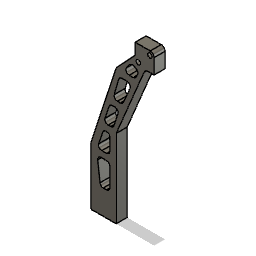
arma_1_(version_minecraft)_v3 (Autodesk Fusion 360 design; units mm, degrees)
Autodesk Fusion 360 part; units mm, degrees
sketch "Boceto1" plane through (0, 0, 0) normal (0, 0, 1) x (1, 0, 0)
sketch "Boceto2" plane through (0, 0, 0) normal (0, 0, 1) x (1, 0, 0)
  line L0 (0, 0) -> (0, 77.2995)
  line L1 (0, 77.2995) -> (40, 200)
  line L2 (40, 200) -> (77.2455, 240)
  line L3 (77.2455, 240) -> (94.1667, 240)
  line L4 (94.1667, 240) -> (40, 110)
  line L5 (40, 110) -> (40, 0)
  line L6 (40, 0) -> (0, 0)
  line L7 (73, 230) -> (85, 230)
  line L8 (85, 230) -> (70, 200)
  line L9 (70, 200) -> (50, 200)
  line L10 (50, 200) -> (73, 230)
  line L11 (45, 190) -> (65, 190)
  line L12 (65, 190) -> (50, 155)
  line L13 (50, 155) -> (35, 155)
  line L14 (35, 155) -> (45, 190)
  line L15 (30, 145) -> (45, 145)
  line L16 (45, 145) -> (35, 115)
  line L17 (35, 115) -> (20, 115)
  line L18 (20, 115) -> (30, 145)
  line L19 (20, 105) -> (30, 105)
  line L20 (30, 105) -> (30, 75)
  line L21 (30, 75) -> (10, 75)
  line L22 (10, 75) -> (20, 105)
  line L23 (10, 65) -> (30, 65)
  line L24 (30, 65) -> (30, 25)
  line L25 (30, 25) -> (15, 25)
  line L26 (15, 25) -> (10, 65)
  constraint coincident L0.start L6.end
  constraint vertical L0
  constraint perpendicular L0 L3
  constraint vertical L5
  constraint perpendicular L0 L6
  constraint horizontal L7
  constraint parallel L7 L9
  constraint horizontal L11
  constraint parallel L11 L13
  constraint horizontal L15
  constraint parallel L15 L17
  constraint parallel L16 L18
  constraint horizontal L19
  constraint perpendicular L19 L20
  constraint perpendicular L20 L21
  constraint horizontal L23
  constraint perpendicular L23 L24
  constraint perpendicular L24 L25
extrude "Extruir1" add sketch "Boceto2" along normal blind 10 makes body 1
cylinder "CilindroPrimitivo1" add diameter 47.743 height 10 placed x (1, 0, 0) y (0, 1, 0) z (0, 0, 1) at (20, 10, 10) separate body makes body 2
copy_body "CopiarPegarCuerpos1" bodies 2 makes body 3
move_body "Desplazar1" bodies 3 to x (1, 0, 0) y (0, 1, 0) z (0, 0, 1) at (0, 0, -20)
hole "Agujero1" at (20.2379, 10.8287, -10) direction (0, 0, 1) diameter 20 depth 20 tip angle 118 bodies 1 2 3
hole "Agujero2" at (20, 10, 20) direction (0, 0, -1) diameter 20 depth 20 tip angle 118 bodies 1 2 3
sketch "Boceto4" plane through (0, 0, 0) normal (0, 0, 1) x (1, 0, 0)
sketch "Boceto5" plane through (0, 0, 10) normal (0, 0, 1) x (1, 0, 0)
  arc A0 (10.5162, 13.1713) -> (20, 0) centre (20, 10) ccw
  arc A1 (29.7218, 7.6575) -> (10.5162, 13.1713) centre (20.2379, 10.8287) ccw
  arc A2 (20, 0) -> (29.7218, 7.6575) centre (20, 10) ccw
  line L0 (20, 0) -> (40, 0)
  line L1 (40, 0) -> (40, 110)
  line L2 (40, 110) -> (94.1667, 240)
  line L3 (94.1667, 240) -> (77.2455, 240)
  line L4 (77.2455, 240) -> (40, 200)
  line L5 (40, 200) -> (0, 77.2995)
  line L6 (0, 77.2995) -> (0, 0)
  line L7 (0, 0) -> (20, 0)
  line L8 (70, 200) -> (50, 200)
  line L9 (50, 200) -> (73, 230)
  line L10 (73, 230) -> (85, 230)
  line L11 (85, 230) -> (70, 200)
  line L12 (50, 155) -> (35, 155)
  line L13 (35, 155) -> (45, 190)
  line L14 (45, 190) -> (65, 190)
  line L15 (65, 190) -> (50, 155)
  line L16 (35, 115) -> (20, 115)
  line L17 (20, 115) -> (30, 145)
  line L18 (30, 145) -> (45, 145)
  line L19 (45, 145) -> (35, 115)
  line L20 (30, 75) -> (10, 75)
  line L21 (10, 75) -> (20, 105)
  line L22 (20, 105) -> (30, 105)
  line L23 (30, 105) -> (30, 75)
  line L24 (30, 25) -> (15, 25)
  line L25 (15, 25) -> (10, 65)
  line L26 (10, 65) -> (30, 65)
  line L27 (30, 65) -> (30, 25)
  line L28 (50, 340) -> (50, 330)
  line L29 (50, 330) -> (60, 330)
  line L30 (60, 330) -> (60, 320)
  line L31 (60, 320) -> (100, 320)
  line L32 (100, 320) -> (100, 310)
  line L33 (100, 310) -> (110, 310)
  line L34 (110, 310) -> (110, 300)
  line L35 (110, 300) -> (120, 300)
  line L36 (120, 300) -> (120, 260)
  line L37 (120, 260) -> (130, 260)
  line L38 (130, 260) -> (130, 250)
  line L39 (130, 250) -> (140, 250)
  line L40 (140, 250) -> (140, 260)
  line L41 (140, 260) -> (150, 260)
  line L42 (150, 260) -> (150, 310)
  line L43 (150, 310) -> (140, 310)
  line L44 (140, 310) -> (140, 340)
  line L45 (140, 340) -> (110, 340)
  line L46 (110, 340) -> (110, 350)
  line L47 (110, 350) -> (60, 350)
  line L48 (60, 350) -> (60, 340)
  line L49 (60, 340) -> (50, 340)
  constraint vertical L28
  constraint perpendicular L28 L29
  constraint perpendicular L29 L30
  constraint perpendicular L30 L31
  constraint perpendicular L29 L32
  constraint perpendicular L32 L33
  constraint perpendicular L33 L34
  constraint perpendicular L34 L35
  constraint perpendicular L35 L36
  constraint perpendicular L36 L37
  constraint perpendicular L37 L38
  constraint perpendicular L38 L39
  constraint perpendicular L39 L40
  constraint perpendicular L40 L41
  constraint perpendicular L41 L42
  constraint perpendicular L42 L43
  constraint perpendicular L43 L44
  constraint perpendicular L44 L45
  constraint perpendicular L43 L46
  constraint perpendicular L46 L47
  constraint perpendicular L47 L48
  constraint perpendicular L28 L49
extrude "Extruir2" add sketch "Boceto5" along normal blind 10 separate body contours L28 L29 L30 L31 L32 L33 L34 L35 L36 L37 L38 L39 L40 L41 L42 L43 L44 L45 L46 L47 L48 L49 makes body 4
move_body "Desplazar2" bodies 4 to x (1, 0, 0) y (0, 1, 0) z (0, 0, 1) at (-20.4494, -47.9195, 22.1569)
move_body "Desplazar3" bodies 4 to x (1, 0, 0) y (0, 1, 0) z (0, 0, 1) at (4.6161, -12.0805, -32.1569)
move_body "Desplazar4" bodies 4 to x (1, 0, 0) y (0, 1, 0) z (0, 0, 1) at (0, -10, 0)
box "CajaPrimitiva1" add length 30 width 30 height 10 placed x (0, -1, 0) y (-1, 0, 0) z (0, 0, -1) at (100, 250, 0) separate body makes body 5
box "CajaPrimitiva2" cut length 30 width 30 height 10 placed x (0, -1, 0) y (1, 0, 0) z (0, 0, 1) at (70, 250, 0) bodies 1 4
move_body "Desplazar6" bodies 5 to x (1, 0, 0) y (0, 1, 0) z (0, 0, 1) at (0, 0, 10)
delete_body "QuitarCuerpo1" bodies 2
delete_body "QuitarCuerpo2" bodies 3
scale "Escala1" factor 0.9 about (40, 110, 0) bodies 4 5 1
scale "Escala2" factor 0.8 about (40, 110, 0) bodies 5 4 1
scale "Scale3" factor 0.8 about (40, 110, 0) bodies 5 4 1
copy_body "CopyPasteBodies3" bodies 1 5 4 makes body 6 makes body 7 makes body 8
sketch "Sketch8" plane through (0, 0, 5.76) normal (0, 0, 1) x (1, 0, 0)
  line L0 (42.4, 190.64) -> (74.56, 190.64)
  line L1 (74.56, 190.64) -> (74.56, 179.12)
  line L2 (74.56, 179.12) -> (76.96, 179.12)
  line L3 (76.96, 179.12) -> (76.96, 156.08)
  line L4 (76.96, 156.08) -> (82.72, 156.08)
  line L5 (82.72, 156.08) -> (82.72, 150.32)
  line L6 (82.72, 150.32) -> (88.48, 150.32)
  line L7 (88.48, 150.32) -> (88.48, 156.08)
  line L8 (88.48, 156.08) -> (94.24, 156.08)
  line L9 (94.24, 156.08) -> (94.24, 184.88)
  line L10 (94.24, 184.88) -> (88.48, 184.88)
  line L11 (88.48, 184.88) -> (88.48, 202.16)
  line L12 (88.48, 202.16) -> (71.2, 202.16)
  line L13 (71.2, 202.16) -> (71.2, 207.92)
  line L14 (71.2, 207.92) -> (42.4, 207.92)
  line L15 (42.4, 207.92) -> (42.4, 202.16)
  line L16 (42.4, 202.16) -> (36.64, 202.16)
  line L17 (36.64, 202.16) -> (36.64, 196.4)
  line L18 (36.64, 196.4) -> (42.4, 196.4)
  line L19 (42.4, 196.4) -> (42.4, 190.64)
  line L20 (57.28, 173.36) -> (74.56, 173.36)
  line L21 (74.56, 173.36) -> (74.56, 190.64)
  line L22 (74.56, 190.64) -> (57.28, 190.64)
  line L23 (57.28, 190.64) -> (57.28, 173.36)
  circle A0 centre (62.9785, 200.1725) radius 2
  line L24 (62.9785, 200.1725) -> (84.1917, 178.9593)
  circle A1 centre (84.1917, 178.9593) radius 2
  circle A2 centre (60.1084, 176.1884) radius 2
  line L25 (60.1084, 176.1884) -> (70.715, 186.795)
  circle A3 centre (70.715, 186.795) radius 2
  line L26 (57.28, 173.36) -> (74.56, 190.64) construction
  dimension "d32" = 4
  dimension "d33" = 30
  dimension "d34" = 4
  dimension "d35" = 4
  dimension "d36" = 15
  dimension "d37" = 4
  dimension "d38" = 5
  dimension "d39" = 45
  dimension "d40" = 15
  dimension "d41" = 4
  constraint coincident A0.centre L24.start
  constraint coincident L24.end A1.centre
  constraint coincident A2.centre L25.start
  constraint coincident L25.end A3.centre
  constraint coincident L20.start L23.end
  constraint coincident L0.end L1.start
  constraint collinear L25 L26
  measures "d32" diameter of A0
  measures "d33" distance of A0.centre L24.end
  measures "d34" diameter of A1
  measures "d35" diameter of A2
  measures "d36" distance of A2.centre L25.end
  measures "d37" diameter of A3
  measures "d38" distance of L2.end L24
  measures "d39" angle of L22 L24
  measures "d40" distance of L0.end A0.centre
  measures "d41" distance of A2.centre L20.start
extrude "Extrude3" cut sketch "Sketch8" against normal blind 59 contours A0 | A1 | A2 | A3 bodies 4 5
sketch "Sketch9" plane through (0, 0, 0) normal (0, 0, -1) x (-1, 0, 0)
  line L0 (-37.12, 135.92) -> (-45.76, 135.92)
  line L1 (-45.76, 135.92) -> (-54.4, 156.08)
  line L2 (-54.4, 156.08) -> (-42.88, 156.08)
  line L3 (-42.88, 156.08) -> (-37.12, 135.92)
  line L4 (-28.48, 112.88) -> (-37.12, 112.88)
  line L5 (-37.12, 112.88) -> (-42.88, 130.16)
  line L6 (-42.88, 130.16) -> (-34.24, 130.16)
  line L7 (-34.24, 130.16) -> (-28.48, 112.88)
  line L8 (-22.72, 89.84) -> (-34.24, 89.84)
  line L9 (-34.24, 89.84) -> (-34.24, 107.12)
  line L10 (-34.24, 107.12) -> (-28.48, 107.12)
  line L11 (-28.48, 107.12) -> (-22.72, 89.84)
  line L12 (-25.6, 61.04) -> (-34.24, 61.04)
  line L13 (-34.24, 61.04) -> (-34.24, 84.08)
  line L14 (-34.24, 84.08) -> (-22.72, 84.08)
  line L15 (-22.72, 84.08) -> (-25.6, 61.04)
  line L16 (-63.04, 173.36) -> (-66.4, 173.36)
  line L17 (-66.4, 173.36) -> (-40, 110)
  line L18 (-40, 110) -> (-40, 46.64)
  line L19 (-40, 46.64) -> (-28.48, 46.64)
  arc A0 (-34.0797, 51.0507) -> (-28.48, 46.64) centre (-28.48, 52.4) ccw
  arc A1 (-23.0173, 54.2267) -> (-34.0797, 51.0507) centre (-28.617, 52.8773) ccw
  arc A2 (-28.48, 46.64) -> (-23.0173, 54.2267) centre (-28.48, 52.4) ccw
  line L20 (-28.48, 46.64) -> (-16.96, 46.64)
  line L21 (-16.96, 46.64) -> (-16.96, 91.1645)
  line L22 (-16.96, 91.1645) -> (-40, 161.84)
  line L23 (-40, 161.84) -> (-57.28, 180.398)
  line L24 (-57.28, 180.398) -> (-57.28, 176.8661)
  line L25 (-57.28, 176.8661) -> (-45.76, 161.84)
  line L26 (-45.76, 161.84) -> (-57.28, 161.84)
  line L27 (-57.28, 161.84) -> (-63.04, 173.36)
  line L28 (-60.7894, 168.8589) -> (-53.8148, 172.3462)
  circle A3 centre (-70.715, 186.795) radius 2
  circle A4 centre (-60.1084, 176.1884) radius 2
  line L29 (-74.56, 173.36) -> (-57.28, 173.36)
  line L30 (-57.28, 173.36) -> (-57.28, 190.64)
  line L31 (-57.28, 190.64) -> (-74.56, 190.64)
  line L32 (-74.56, 190.64) -> (-74.56, 173.36)
  constraint coincident L27 L28.start
  constraint coincident L25 L28.end
  constraint perpendicular L27 L28
extrude "Extrude4" add sketch "Sketch9" against normal blind 5.76 contours L25 L27 L28 L29 L30 bodies 5 1
fillet "Fillet1" radius 3 4 edges at (57.28, 161.84, 2.88) (45.76, 161.84, 2.88) (53.8148, 172.3462, 2.88) (60.7894, 168.8589, 2.88) on bodies 5
fillet "Fillet2" radius 4 1 edges at (66.4, 173.36, 2.88) on bodies 5
fillet "Fillet3" radius 3 16 edges at (42.88, 156.08, 2.88) (54.4, 156.08, 2.88) (45.76, 135.92, 2.88) (37.12, 135.92, 2.88) (34.24, 130.16, 2.88) (42.88, 130.16, 2.88) (34.24, 107.12, 2.88) (25.6, 61.04, 2.88) (28.48, 112.88, 2.88) (37.12, 112.88, 2.88) (28.48, 107.12, 2.88) (22.72, 89.84, 2.88) (34.24, 89.84, 2.88) (34.24, 61.04, 2.88) (34.24, 84.08, 2.88) (22.72, 84.08, 2.88) on bodies 5
sketch "Sketch10" plane through (0, 0, 0) normal (0, 0, -1) x (-1, 0, 0)
  arc A0 (-51.8402, 161.84) -> (-49.4594, 166.6653) centre (-51.8402, 164.84) ccw
  line L0 (-51.8402, 161.84) -> (-55.4259, 161.84)
  arc A1 (-58.1092, 163.4984) -> (-55.4259, 161.84) centre (-55.4259, 164.84) ccw
  line L1 (-58.1092, 163.4984) -> (-59.4478, 166.1756)
  arc A2 (-58.1062, 170.2005) -> (-59.4478, 166.1756) centre (-56.7645, 167.5173) ccw
  line L2 (-58.1062, 170.2005) -> (-56.0302, 171.2385)
  arc A3 (-52.3077, 170.3805) -> (-56.0302, 171.2385) centre (-54.6886, 168.5552) ccw
  line L3 (-52.3077, 170.3805) -> (-49.4594, 166.6653)
  arc A4 (-34.24, 64.04) -> (-31.24, 61.04) centre (-31.24, 64.04) ccw
  line L4 (-34.24, 64.04) -> (-34.24, 81.08)
  arc A5 (-31.24, 84.08) -> (-34.24, 81.08) centre (-31.24, 81.08) ccw
  line L5 (-31.24, 84.08) -> (-26.1183, 84.08)
  arc A6 (-23.1415, 80.7079) -> (-26.1183, 84.08) centre (-26.1183, 81.08) ccw
  line L6 (-23.1415, 80.7079) -> (-25.2715, 63.6679)
  arc A7 (-28.2483, 61.04) -> (-25.2715, 63.6679) centre (-28.2483, 64.04) ccw
  line L7 (-28.2483, 61.04) -> (-31.24, 61.04)
  arc A8 (-34.24, 92.84) -> (-31.24, 89.84) centre (-31.24, 92.84) ccw
  line L8 (-34.24, 92.84) -> (-34.24, 104.12)
  arc A9 (-31.24, 107.12) -> (-34.24, 104.12) centre (-31.24, 104.12) ccw
  line L9 (-31.24, 107.12) -> (-30.6423, 107.12)
  arc A10 (-27.7962, 105.0687) -> (-30.6423, 107.12) centre (-30.6423, 104.12) ccw
  line L10 (-27.7962, 105.0687) -> (-24.0362, 93.7887)
  arc A11 (-26.8823, 89.84) -> (-24.0362, 93.7887) centre (-26.8823, 92.84) ccw
  line L11 (-26.8823, 89.84) -> (-31.24, 89.84)
  arc A12 (-37.8038, 114.9313) -> (-34.9577, 112.88) centre (-34.9577, 115.88) ccw
  line L12 (-37.8038, 114.9313) -> (-41.5638, 126.2113)
  arc A13 (-38.7177, 130.16) -> (-41.5638, 126.2113) centre (-38.7177, 127.16) ccw
  line L13 (-38.7177, 130.16) -> (-36.4023, 130.16)
  arc A14 (-33.5562, 128.1087) -> (-36.4023, 130.16) centre (-36.4023, 127.16) ccw
  line L14 (-33.5562, 128.1087) -> (-29.7962, 116.8287)
  arc A15 (-32.6423, 112.88) -> (-29.7962, 116.8287) centre (-32.6423, 115.88) ccw
  line L15 (-32.6423, 112.88) -> (-34.9577, 112.88)
  arc A16 (-46.5392, 137.7382) -> (-43.7818, 135.92) centre (-43.7818, 138.92) ccw
  line L16 (-46.5392, 137.7382) -> (-52.6078, 151.8982)
  arc A17 (-49.8504, 156.08) -> (-52.6078, 151.8982) centre (-49.8504, 153.08) ccw
  line L17 (-49.8504, 156.08) -> (-45.1429, 156.08)
  arc A18 (-42.2583, 153.9042) -> (-45.1429, 156.08) centre (-45.1429, 153.08) ccw
  line L18 (-42.2583, 153.9042) -> (-38.2126, 139.7442)
  arc A19 (-41.0972, 135.92) -> (-38.2126, 139.7442) centre (-41.0972, 138.92) ccw
  line L19 (-41.0972, 135.92) -> (-43.7818, 135.92)
  circle A20 centre (-70.715, 186.795) radius 2
  circle A21 centre (-60.1084, 176.1884) radius 2
  line L20 (-65.3744, 170.8985) -> (-40, 110)
  line L21 (-40, 110) -> (-40, 46.64)
  line L22 (-40, 46.64) -> (-28.48, 46.64)
  arc A22 (-34.0797, 51.0507) -> (-28.48, 46.64) centre (-28.48, 52.4) ccw
  arc A23 (-23.0173, 54.2267) -> (-34.0797, 51.0507) centre (-28.617, 52.8773) ccw
  arc A24 (-28.48, 46.64) -> (-23.0173, 54.2267) centre (-28.48, 52.4) ccw
  line L23 (-28.48, 46.64) -> (-16.96, 46.64)
  line L24 (-16.96, 46.64) -> (-16.96, 91.1645)
  line L25 (-16.96, 91.1645) -> (-40, 161.84)
  line L26 (-40, 161.84) -> (-57.28, 180.398)
  line L27 (-57.28, 180.398) -> (-57.28, 190.64)
  line L28 (-57.28, 190.64) -> (-74.56, 190.64)
  line L29 (-74.56, 190.64) -> (-74.56, 173.36)
  line L30 (-74.56, 173.36) -> (-69.0667, 173.36)
  arc A25 (-65.3744, 170.8985) -> (-69.0667, 173.36) centre (-69.0667, 169.36) ccw
  line L31 (-40, 46.64) -> (-16.96, 46.64)
  line L32 (-16.96, 46.64) -> (-16.96, 38.64)
  line L33 (-16.96, 38.64) -> (-40, 38.64)
  line L34 (-40, 38.64) -> (-40, 46.64)
  dimension "d52" = 8
  constraint horizontal L31
  constraint vertical L32
  constraint horizontal L33
  constraint vertical L34
  constraint coincident L21.end L22.start
  constraint collinear L24 L32
  measures "d52" distance of L21.end L33.end
extrude "Extrude5" add sketch "Sketch10" against normal blind 5.76 contours L22 L23 L31 L32 L33 L34 bodies 5
delete_body "RemoveBody3" bodies 6
delete_body "RemoveBody4" bodies 7
delete_body "RemoveBody5" bodies 8
copy_body "Body->Comp1" bodies 4 removing the originals makes body 9 in component "Component"
copy_body "Body->Comp2" bodies 5 removing the originals makes body 10 in component "Component'"
move_face "OffsetFaces1" offset 4.24 1 faces at (83.84, 192.56, 0) on bodies 9 in component "Component"
move_face "OffsetFaces1'" offset 4.24 1 faces at (28.5066, 41.3069, 0) on bodies 10 in component "Component'"
sketch "Sketch11" plane through (0, 0, 5.76) normal (0, 0, 1) x (1, 0, 0)
  arc A0 (23.0173, 54.2267) -> (34.0797, 51.0507) centre (28.48, 52.4) ccw
  arc A1 (34.0797, 51.0507) -> (23.0173, 54.2267) centre (28.617, 52.8773) ccw
  line L0 (16.96, 91.1645) -> (16.96, 38.64)
  line L1 (16.96, 38.64) -> (40, 38.64)
  line L2 (40, 38.64) -> (40, 110)
  line L3 (40, 110) -> (65.3744, 170.8985)
  arc A2 (69.0667, 173.36) -> (65.3744, 170.8985) centre (69.0667, 169.36) ccw
  line L4 (69.0667, 173.36) -> (74.56, 173.36)
  line L5 (74.56, 173.36) -> (74.56, 190.64)
  line L6 (74.56, 190.64) -> (57.28, 190.64)
  line L7 (57.28, 190.64) -> (57.28, 180.398)
  line L8 (57.28, 180.398) -> (40, 161.84)
  line L9 (40, 161.84) -> (16.96, 91.1645)
  line L10 (31.24, 61.04) -> (28.2483, 61.04)
  arc A3 (25.2715, 63.6679) -> (28.2483, 61.04) centre (28.2483, 64.04) ccw
  line L11 (25.2715, 63.6679) -> (23.1415, 80.7079)
  arc A4 (26.1183, 84.08) -> (23.1415, 80.7079) centre (26.1183, 81.08) ccw
  line L12 (26.1183, 84.08) -> (31.24, 84.08)
  arc A5 (34.24, 81.08) -> (31.24, 84.08) centre (31.24, 81.08) ccw
  line L13 (34.24, 81.08) -> (34.24, 64.04)
  arc A6 (31.24, 61.04) -> (34.24, 64.04) centre (31.24, 64.04) ccw
  line L14 (31.24, 89.84) -> (26.8823, 89.84)
  arc A7 (24.0362, 93.7887) -> (26.8823, 89.84) centre (26.8823, 92.84) ccw
  line L15 (24.0362, 93.7887) -> (27.7962, 105.0687)
  arc A8 (30.6423, 107.12) -> (27.7962, 105.0687) centre (30.6423, 104.12) ccw
  line L16 (30.6423, 107.12) -> (31.24, 107.12)
  arc A9 (34.24, 104.12) -> (31.24, 107.12) centre (31.24, 104.12) ccw
  line L17 (34.24, 104.12) -> (34.24, 92.84)
  arc A10 (31.24, 89.84) -> (34.24, 92.84) centre (31.24, 92.84) ccw
  line L18 (34.9577, 112.88) -> (32.6423, 112.88)
  arc A11 (29.7962, 116.8287) -> (32.6423, 112.88) centre (32.6423, 115.88) ccw
  line L19 (29.7962, 116.8287) -> (33.5562, 128.1087)
  arc A12 (36.4023, 130.16) -> (33.5562, 128.1087) centre (36.4023, 127.16) ccw
  line L20 (36.4023, 130.16) -> (38.7177, 130.16)
  arc A13 (41.5638, 126.2113) -> (38.7177, 130.16) centre (38.7177, 127.16) ccw
  line L21 (41.5638, 126.2113) -> (37.8038, 114.9313)
  arc A14 (34.9577, 112.88) -> (37.8038, 114.9313) centre (34.9577, 115.88) ccw
  line L22 (43.7818, 135.92) -> (41.0972, 135.92)
  arc A15 (38.2126, 139.7442) -> (41.0972, 135.92) centre (41.0972, 138.92) ccw
  line L23 (38.2126, 139.7442) -> (42.2583, 153.9042)
  arc A16 (45.1429, 156.08) -> (42.2583, 153.9042) centre (45.1429, 153.08) ccw
  line L24 (45.1429, 156.08) -> (49.8504, 156.08)
  arc A17 (52.6078, 151.8982) -> (49.8504, 156.08) centre (49.8504, 153.08) ccw
  line L25 (52.6078, 151.8982) -> (46.5392, 137.7382)
  arc A18 (43.7818, 135.92) -> (46.5392, 137.7382) centre (43.7818, 138.92) ccw
  circle A19 centre (70.715, 186.795) radius 2
  circle A20 centre (60.1084, 176.1884) radius 2
  line L26 (59.4478, 166.1756) -> (58.1092, 163.4984)
  arc A21 (55.4259, 161.84) -> (58.1092, 163.4984) centre (55.4259, 164.84) ccw
  line L27 (55.4259, 161.84) -> (51.8402, 161.84)
  arc A22 (49.4594, 166.6653) -> (51.8402, 161.84) centre (51.8402, 164.84) ccw
  line L28 (49.4594, 166.6653) -> (52.3077, 170.3805)
  arc A23 (56.0302, 171.2385) -> (52.3077, 170.3805) centre (54.6886, 168.5552) ccw
  line L29 (56.0302, 171.2385) -> (58.1062, 170.2005)
  arc A24 (59.4478, 166.1756) -> (58.1062, 170.2005) centre (56.7645, 167.5173) ccw
extrude "Extrude1" add sketch "Sketch11" against normal blind 10 contours A0 A1 bodies 10 in component "Component'"
fillet "Fillet1'" radius 3 7 edges at (82.72, 156.08, 0.76) (88.48, 156.08, 0.76) (42.4, 196.4, 0.76) (42.4, 202.16, 0.76) (71.2, 202.16, 0.76) (88.48, 184.88, 0.76) (76.96, 179.12, 0.76) on bodies 9 in component "Component"
fillet "Fillet2'" radius 3.5 1 edges at (74.56, 190.64, 0.76) on bodies 9 in component "Component"
fillet "Fillet1''" radius 3.5 1 edges at (74.56, 190.64, 0.76) on bodies 10 in component "Component'"
component "Component" placed x (1, 0, 0) y (0, 1, 0) z (0, 0, 1) at (0, 0, 0)
component "Component'" placed x (1, 0, 0) y (0, 1, 0) z (0, 0, 1) at (0, 0, 0)
equation "d40 = d33 / 2"
